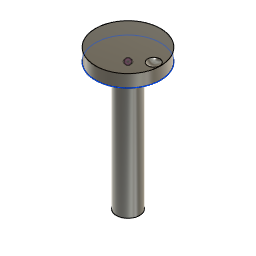
Hand_Crank_Affector_3D_Prints_v1 (Autodesk Fusion 360 design; units mm, degrees)
Autodesk Fusion 360 part; units mm, degrees
sketch "Sketch1" plane through (0, 0, 0) normal (0, 0, 1) x (1, 0, 0)
  circle A0 centre (0, 0) radius 10.75
  dimension "d1" = 21.5
  constraint coincident A0.centre origin
  measures "d1" diameter of A0
extrude "Extrude1" add sketch "Sketch1" along normal blind 114 makes body 1
sketch "Sketch2" plane through (0, 0, 114) normal (0, 0, 1) x (-1, 0, 0)
  circle A0 centre (0, 0) radius 10.75
  circle A1 centre (0, 0) radius 9.75
  dimension "d6" = 19.5
  constraint concentric A0 A1
  measures "d6" diameter of A1
extrude "Extrude2" cut sketch "Sketch2" against normal blind 2.5 contours A1 bodies 1
copy_body "CutPasteBodies1" bodies 1 removing the originals makes body 2 in component "Main Housing"
sketch "Sketch1 (2)" plane through (0, 0, 111.5) normal (0, 0, 1) x (-1, 0, 0) in component "Main Housing"
  circle A0 centre (0, 0) radius 9.75
  line L0 (7.3121, 6.4494) -> (7.3121, -6.4494)
  line L1 (7, -10.4909) -> (-7, 10.4909) construction
  line L2 (-7, -10.4909) -> (7, 10.4909) construction
  circle A1 centre (0, 0) radius 8.75
  circle A2 centre (6.25, 0) radius 2.5
  line L3 (7.3121, 0) -> (6.25, 0) construction
  line L4 (0, -8.75) -> (0, 8.75) construction
  circle A3 centre (-6.25, 0) radius 2.5
  line L5 (-7.3121, 6.4494) -> (-7.3121, -6.4494)
  dimension "d9" = 14
  dimension "d14" = 5
  dimension "d15" = 17.5
  constraint coincident L1 A0.centre
  constraint coincident L2 A0.centre
  constraint coincident A0.centre A1.centre
  constraint coincident A0 L0.end
  constraint coincident A0 L0.start
  constraint midpoint L0 L3.start
  constraint coincident A2.centre L3.end
  constraint perpendicular L0 L3
  constraint tangent A1 A2
  constraint coincident A1 L4.start
  constraint coincident A1 L4.end
  constraint vertical L4
  constraint symmetric A2 L4 A3
  constraint symmetric L0.end L4 L5.end
  constraint symmetric L0.start L4 L5.start
  measures "d9" distance of L1.end L2.end
  measures "d14" diameter of A2
  measures "d15" diameter of A1
extrude "Extrude1'" cut sketch "Sketch1 (2)" against normal up to surface (111.5 mm away) contours L0 A1 A2 | L0 A1 A2 | A1 A3 L5 | L0 A2 | L0 A2 | A1 A3 L5 | A3 L5 | A3 L5 bodies 2 in component "Main Housing"
extrude "Extrude4" cut sketch "Sketch1 (2)" against normal blind 9 contours L0 A1 A2 A3 L5 | A1 A3 L5 | A1 A3 L5 | A3 L5 | A3 L5 bodies 2 in component "Main Housing"
sketch "Sketch2 (2)" plane through (0, 0, 111.5) normal (0, 0, 1) x (-1, 0, 0) in component "Main Housing"
  line L0 (-4, -7.7822) -> (-4, 7.7822)
  line L1 (4, 7.7822) -> (4, -7.7822)
  line L2 (4, -12.291) -> (-4, 12.291) construction
  line L3 (-4, -12.291) -> (4, 12.291) construction
  circle A0 centre (0, 0) radius 8.75
  circle A1 centre (0, 0) radius 8.75
  line L4 (-4, -6.75) -> (4, -6.75)
  line L5 (4, -6.75) -> (4, 6.75)
  line L6 (4, 6.75) -> (-4, 6.75)
  line L7 (-4, 6.75) -> (-4, -6.75)
  line L8 (-4, -6.75) -> (4, 6.75) construction
  line L9 (4, -6.75) -> (-4, 6.75) construction
  dimension "d21" = 8
  dimension "d22" = 13.5
  constraint parallel L0 L1
  constraint coincident L2 A0.centre
  constraint coincident L3 A0.centre
  constraint coincident A0.centre A1.centre
  constraint perpendicular L4 L5
  constraint parallel L4 L6
  constraint parallel L5 L7
  constraint horizontal L4
  constraint coincident L8 A0.centre
  constraint coincident L9 A0.centre
  constraint coincident A0 L1.start
  constraint coincident A0 L0.end
  constraint coincident A0 L0.start
  constraint coincident A0 L1.end
  measures "d21" distance of L2.end L3.end
  measures "d22" distance of L4.end L5.end
extrude "Extrude5" add sketch "Sketch2 (2)" against normal up to surface (9 mm away) contours L0 L1 A0 A1 L4 | L0 L1 A0 A1 L6 bodies 2 in component "Main Housing"
sketch "Sketch1 (3)" plane through (0, 0, 111.5) normal (0, 0, 1) x (-1, 0, 0) in component "Cover"
  circle A0 centre (0, 0) radius 9.75
  arc A1 (-4, 7.7822) -> (-4, -7.7822) centre (0, 0) ccw
  line L0 (-4, 7.7822) -> (-4, 6.75)
  line L1 (-4, 6.75) -> (4, 6.75)
  line L2 (4, 6.75) -> (4, 7.7822)
  arc A2 (4, -7.7822) -> (4, 7.7822) centre (0, 0) ccw
  line L3 (4, -7.7822) -> (4, -6.75)
  line L4 (4, -6.75) -> (-4, -6.75)
  line L5 (-4, -6.75) -> (-4, -7.7822)
  circle A3 centre (0, 0) radius 9.75
  circle A4 centre (0, 0) radius 9.65
  circle A5 centre (0, 0) radius 4.25
  dimension "d54" = -0.1
  dimension "d55" = 8.5
  constraint concentric A0 A3
  constraint concentric A3 A5
  measures "d55" diameter of A5
extrude "Extrude1''" add sketch "Sketch1 (3)" along normal up to surface (2.5 mm away) separate body contours A1 L0 L1 L2 A2 L3 L4 L5 | A4 makes body 3 in component "Cover"
sketch "Sketch1 (4)" plane through (0, 0, 0) normal (0, 0, 1) x (1, 0, 0) in component "HandCrank"
  circle A0 centre (0, 0) radius 3.3
  line L0 (0, 0) -> (3.3, 0) construction
  line L1 (0, 3.3) -> (0, 0) construction
  line L2 (-3.0741, -1.2) -> (3.0741, -1.2)
  circle A1 centre (0, 0) radius 30
  dimension "d61" = 6.6
  dimension "d62" = 4.5
  dimension "d71" = 60
  constraint coincident A0.centre L0.start
  constraint coincident A0 L0.end
  constraint horizontal L0
  constraint coincident A0 L1.start
  constraint perpendicular L0 L1
  constraint parallel L0 L2
  constraint coincident A0 L2.end
  constraint coincident A0 L2.start
  measures "d61" diameter of A0
  measures "d62" distance of L1.start L2
  measures "d71" diameter of A1
extrude "Extrude8" add sketch "Sketch1 (4)" along normal blind 2.5 separate body makes body 4 in component "HandCrank"
extrude "Extrude9" add sketch "Sketch1 (4)" along normal blind 7 from surface at 2.5 contours A0 L2 | A1 picked at (-0.7491, -1.6055) bodies 4 in component "HandCrank"
sketch "Sketch9" plane through (0, 0, 9.5) normal (0, 0, 1) x (-1, 0, 0) in component "HandCrank"
  arc A0 (-3.0741, 1.2) -> (3.0741, 1.2) centre (0, 0) ccw
  line L0 (-3.0741, 1.2) -> (3.0741, 1.2)
  circle A1 centre (0, 0) radius 30
  circle A2 centre (0, 0) radius 30
  constraint coincident A0.centre A1.centre
extrude "Extrude10" add sketch "Sketch9" along normal blind 2 contours A0 L0 | A1 A2 bodies 4 in component "HandCrank"
sketch "Sketch10" plane through (0, 0, 0) normal (0, 0, 1) x (1, 0, 0) in component "HandCrank"
  circle A0 centre (0, 0) radius 10.5
  circle A1 centre (0, 0) radius 9
  dimension "d97" = 21
  dimension "d98" = -1.5
  constraint coincident A0.centre A1.centre
  measures "d97" diameter of A0
extrude "Extrude11" add sketch "Sketch10" against normal blind 3.25 bodies 4 in component "HandCrank"
ref_plane "WorkPlane5" through (0, 0, 16.5) normal (0, 0, 1) x (-1, 0, 0) in component "HandCrank"
sphere "SpherePrimitive3" cut diameter 15 placed x (1, 0, 0) y (0, 1, 0) z (0, 0, 1) at (24.003, -0.1719, 16.5) bodies 4 in component "HandCrank"
sketch "Sketch1 (5)" plane through (0, 0, 114) normal (0, 0, 1) x (-1, 0, 0) in component "Cap"
  circle A0 centre (0, 0) radius 9.75
  circle A1 centre (0, 0) radius 10.75
  circle A2 centre (0, 0) radius 9.65
  circle A3 centre (0, 0) radius 3
  dimension "d25" = 19.3
  dimension "d28" = 6
  constraint coincident A0.centre A1.centre
  measures "d25" diameter of A2
  measures "d28" diameter of A3
extrude "Extrude1'''" [suppressed] in component "Cap"
sketch "Sketch1 (6)" plane through (0, 0, 0) normal (0, 0, 1) x (1, 0, 0) in component "Handle"
  circle A0 centre (0, 0) radius 6
  circle A1 centre (-73.0625, 16.9375) radius 4
  line L0 (-72.2634, 20.8568) -> (1.1986, 5.8791)
  line L1 (-74.0694, 13.0663) -> (-1.5104, -5.8068)
  circle A2 centre (0, 0) radius 3
  line L2 (-2.901, -0.7643) -> (2.1609, -2.081)
  line L3 (-0.37, -1.4227) -> (0.7552, 2.9034) construction
  dimension "d41" = 12
  dimension "d42" = 8
  dimension "d43" = 75
  dimension "d44" = 6
  dimension "d48" = 4.47
  constraint coincident A0.centre A2.centre
  constraint tangent A0 L0
  constraint tangent A1 L0
  constraint tangent A1 L1
  constraint tangent A0 L1
  constraint coincident A0 L0.end
  constraint coincident A0 L1.end
  constraint coincident A1 L1.start
  constraint coincident A1 L0.start
  constraint concentric A0 A2
  constraint coincident A2 L2.end
  constraint coincident A2 L2.start
  constraint parallel L1 L2
  constraint midpoint L2 L3.start
  constraint coincident A2 L3.end
  constraint perpendicular L2 L3
  measures "d41" diameter of A0
  measures "d42" diameter of A1
  measures "d43" distance of A0.centre A1.centre
  measures "d44" diameter of A2
  measures "d48" distance of L3.start L3.end
extrude "Extrude1''''" [suppressed] in component "Handle"
extrude "Extrude2'" [suppressed] in component "Handle"
component "Main Housing" placed x (1, 0, 0) y (0, 1, 0) z (0, 0, 1) at (0, 0, 0)
component "Cover" placed x (1, 0, 0) y (0, 1, 0) z (0, 0, 1) at (0, 0, 0)
component "HandCrank" placed x (1, 0, 0) y (0, 1, 0) z (0, 0, 1) at (0, 0, 118)
equation "d1 = diameter"
equation "d2 = length"
equation "diameter = 21.5 mm"
equation "length = 114 mm"
equation "d6 = diameter - 2 mm"
equation "d15 = diameter - 4 mm"
equation "d25 = diameter - 2.2 mm"
named bodies: "Test 1", "Main Body"
